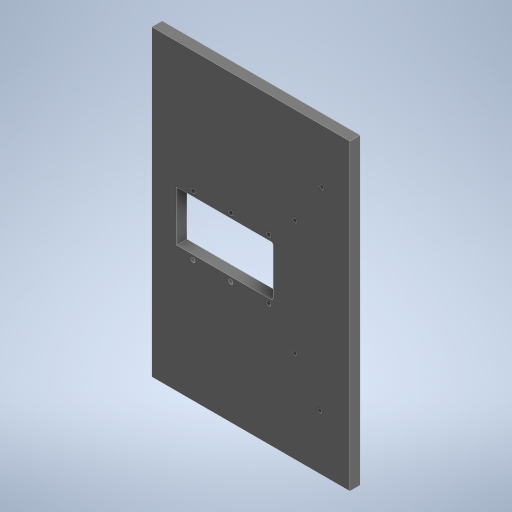
# Autodesk Inventor part: 12_CPY
Saved by Autodesk Inventor 2024.3 (Build 283343000, 343)
## iProperties
Created: 2024-09-08
Part Number: 12_CPY
Material: 아크릴, 선명
Document SubType Name: Modeling
Designer: 구지현
Mass: 132.436 g
Surface Area: 421.006 cm^2
Volume: 111.29 cm^3
Density: 1.19 g/cm^3
Appearance: 회색
Author: 구지현
Autodesk Inventor part; units mm, degrees
ref_plane "YZ Plane" through (0, 0, 0) normal (1, 0, 0) x (0, 1, 0)
ref_plane "XZ Plane" through (0, 0, 0) normal (0, 1, 0) x (-1, 0, 0)
ref_plane "XY Plane" through (0, 0, 0) normal (0, 0, 1) x (1, 0, 0)
ref_plane "작업 평면1" through (-11.501, -90.6951, 25.5) normal (0, 0, 1) x (0, 1, 0)
sketch "스케치1" plane through (-11.501, -90.6951, 25.5) normal (0, 0, 1) x (0, 1, 0)
  line L0 (-0.0049, 0) -> (27.5951, 0)
  line L1 (27.5951, 0) -> (27.5951, 6)
  line L2 (-0.0049, 6) -> (27.5951, 6)
  line L3 (-0.0049, 0) -> (-0.0049, 6)
  line L4 (127.3951, 6) -> (99.7951, 6)
  line L5 (99.7951, 6) -> (99.7951, 0)
  line L6 (127.3951, 0) -> (99.7951, 0)
  line L7 (127.3951, 6) -> (127.3951, 0)
  line L8 (99.8951, -54.101) -> (127.4951, -54.101)
  line L9 (127.4951, -54.101) -> (127.4951, -48.101)
  line L10 (99.8951, -48.101) -> (127.4951, -48.101)
  line L11 (99.8951, -54.101) -> (99.8951, -48.101)
  line L12 (27.4951, -48.101) -> (-0.1049, -48.101)
  line L13 (-0.1049, -48.101) -> (-0.1049, -54.101)
  line L14 (27.4951, -54.101) -> (-0.1049, -54.101)
  line L15 (27.4951, -48.101) -> (27.4951, -54.101)
  line L16 (-0.2463, -60.601) -> (-0.2463, -62.601)
  line L17 (-0.2463, -62.601) -> (1.1951, -62.601)
  line L18 (1.1951, -62.601) -> (1.1951, -92.601)
  line L19 (1.1951, -92.601) -> (-0.2463, -92.601)
  line L20 (-0.2463, -92.601) -> (-0.2463, -94.601)
  line L21 (-0.2463, -94.601) -> (6.0451, -94.601)
  line L22 (21.3451, -94.601) -> (6.0451, -94.601)
  line L23 (21.3451, -94.601) -> (27.6365, -94.601)
  line L24 (27.6365, -92.601) -> (27.6365, -94.601)
  line L25 (27.6365, -92.601) -> (26.1951, -92.601)
  line L26 (26.1951, -62.601) -> (26.1951, -92.601)
  line L27 (26.1951, -62.601) -> (27.6365, -62.601)
  line L28 (27.6365, -60.601) -> (27.6365, -62.601)
  line L29 (27.6365, -60.601) -> (26.6951, -60.601)
  line L30 (26.6951, -60.601) -> (26.6951, -59.101)
  line L31 (0.6951, -59.101) -> (26.6951, -59.101)
  line L32 (0.6951, -59.101) -> (0.6951, -60.601)
  line L33 (0.6951, -60.601) -> (-0.2463, -60.601)
  line L34 (35.6951, -14.501) -> (35.6951, -37.501)
  line L35 (35.6951, -14.501) -> (30.6951, -14.501)
  line L36 (30.6951, -14.501) -> (30.6951, -11.001)
  line L37 (28.6951, -11.001) -> (30.6951, -11.001)
  line L38 (28.6951, -11.001) -> (28.6951, -13.501)
  line L39 (28.6951, -13.501) -> (-1.3049, -13.501)
  line L40 (-1.3049, -13.501) -> (-1.3049, -11.001)
  line L41 (-1.3049, -11.001) -> (-3.3049, -11.001)
  line L42 (-3.3049, -11.001) -> (-3.3049, -16.751)
  line L43 (-5.8049, -16.751) -> (-3.3049, -16.751)
  spline S0 degree 3 poles (-5.8049, -16.751) (-6.0293, -16.751) (-6.2964, -16.7855) (-6.6655, -16.908) (-6.8416, -16.9972) (-7.0685, -17.1834) (-7.1685, -17.3017) (-7.2736, -17.5152) (-7.3049, -17.6421) (-7.3049, -17.751) knots 0 0 0 0 0.358 0.358 0.620378 0.620378 0.826274 0.826274 1 1 1 1
  line L44 (-7.3049, -34.251) -> (-7.3049, -17.751)
  spline S1 degree 3 poles (-7.3049, -34.251) (-7.3049, -34.3599) (-7.2736, -34.4868) (-7.1685, -34.7003) (-7.0685, -34.8186) (-6.8416, -35.0048) (-6.6655, -35.094) (-6.2964, -35.2165) (-6.0293, -35.251) (-5.8049, -35.251) knots 0 0 0 0 0.173726 0.173726 0.379622 0.379622 0.642 0.642 1 1 1 1
  line L45 (-5.8049, -35.251) -> (-3.3049, -35.251)
  line L46 (-3.3049, -35.251) -> (-3.3049, -41.001)
  line L47 (-1.3049, -41.001) -> (-3.3049, -41.001)
  line L48 (-1.3049, -41.001) -> (-1.3049, -38.501)
  line L49 (28.6951, -38.501) -> (-1.3049, -38.501)
  line L50 (28.6951, -38.501) -> (28.6951, -41.001)
  line L51 (28.6951, -41.001) -> (30.6951, -41.001)
  line L52 (30.6951, -41.001) -> (30.6951, -37.501)
  line L53 (35.6951, -37.501) -> (30.6951, -37.501)
  line L54 (135.6951, -14.501) -> (135.6951, -37.501)
  line L55 (135.6951, -14.501) -> (130.6951, -14.501)
  line L56 (130.6951, -14.501) -> (130.6951, -11.001)
  line L57 (128.6951, -11.001) -> (130.6951, -11.001)
  line L58 (128.6951, -11.001) -> (128.6951, -13.501)
  line L59 (128.6951, -13.501) -> (98.6951, -13.501)
  line L60 (98.6951, -13.501) -> (98.6951, -11.001)
  line L61 (98.6951, -11.001) -> (96.6951, -11.001)
  line L62 (96.6951, -11.001) -> (96.6951, -16.751)
  line L63 (94.1951, -16.751) -> (96.6951, -16.751)
  spline S2 degree 3 poles (94.1951, -16.751) (93.9707, -16.751) (93.7036, -16.7855) (93.3345, -16.908) (93.1584, -16.9972) (92.9315, -17.1834) (92.8315, -17.3017) (92.7264, -17.5152) (92.6951, -17.6421) (92.6951, -17.751) knots 0 0 0 0 0.358 0.358 0.620378 0.620378 0.826274 0.826274 1 1 1 1
  line L64 (92.6951, -34.251) -> (92.6951, -17.751)
  spline S3 degree 3 poles (92.6951, -34.251) (92.6951, -34.3599) (92.7264, -34.4868) (92.8315, -34.7003) (92.9315, -34.8186) (93.1584, -35.0048) (93.3345, -35.094) (93.7036, -35.2165) (93.9707, -35.251) (94.1951, -35.251) knots 0 0 0 0 0.173726 0.173726 0.379622 0.379622 0.642 0.642 1 1 1 1
  line L65 (94.1951, -35.251) -> (96.6951, -35.251)
  line L66 (96.6951, -35.251) -> (96.6951, -41.001)
  line L67 (98.6951, -41.001) -> (96.6951, -41.001)
  line L68 (98.6951, -41.001) -> (98.6951, -38.501)
  line L69 (128.6951, -38.501) -> (98.6951, -38.501)
  line L70 (128.6951, -38.501) -> (128.6951, -41.001)
  line L71 (128.6951, -41.001) -> (130.6951, -41.001)
  line L72 (130.6951, -41.001) -> (130.6951, -37.501)
  line L73 (135.6951, -37.501) -> (130.6951, -37.501)
  line L74 (99.7537, -60.601) -> (99.7537, -62.601)
  line L75 (99.7537, -62.601) -> (101.1951, -62.601)
  line L76 (101.1951, -62.601) -> (101.1951, -92.601)
  line L77 (101.1951, -92.601) -> (99.7537, -92.601)
  line L78 (99.7537, -92.601) -> (99.7537, -94.601)
  line L79 (99.7537, -94.601) -> (106.0451, -94.601)
  line L80 (121.3451, -94.601) -> (106.0451, -94.601)
  line L81 (121.3451, -94.601) -> (127.6365, -94.601)
  line L82 (127.6365, -92.601) -> (127.6365, -94.601)
  line L83 (127.6365, -92.601) -> (126.1951, -92.601)
  line L84 (126.1951, -62.601) -> (126.1951, -92.601)
  line L85 (126.1951, -62.601) -> (127.6365, -62.601)
  line L86 (127.6365, -60.601) -> (127.6365, -62.601)
  line L87 (127.6365, -60.601) -> (126.6951, -60.601)
  line L88 (126.6951, -60.601) -> (126.6951, -59.101)
  line L89 (100.6951, -59.101) -> (126.6951, -59.101)
  line L90 (100.6951, -59.101) -> (100.6951, -60.601)
  line L91 (100.6951, -60.601) -> (99.7537, -60.601)
  line L92 (21.3451, 6) -> (21.3451, 12)
  line L93 (1.1951, -62.601) -> (1.1951, 11.399)
  line L94 (-24.3049, -26.001) -> (-24.3049, -76.001)
  line L95 (-24.3049, -76.001) -> (-18.3049, -76.001)
  line L96 (-18.3049, -26.001) -> (-18.3049, -76.001)
  line L97 (-24.3049, -26.001) -> (-18.3049, -26.001)
  line L98 (145.6951, -26.001) -> (145.6951, -76.001)
  line L99 (145.6951, -76.001) -> (151.6951, -76.001)
  line L100 (151.6951, -26.001) -> (151.6951, -76.001)
  line L101 (145.6951, -26.001) -> (151.6951, -26.001)
  line L102 (-24.3049, -52.5323) -> (151.6951, -52.5323)
  line L103 (1.1951, 11.399) -> (-33.5056, 11.399)
  line L104 (1.1951, -62.601) -> (-24.3049, -62.601)
  line L105 (-24.3049, -62.601) -> (151.6951, -62.601)
  line L106 (151.6951, -62.601) -> (151.6951, 11.399)
  line L107 (151.6951, 11.399) -> (-24.3049, 11.399)
  line L108 (-24.3049, 11.399) -> (-24.3049, -62.601)
  circle A0 centre (-0.0049, 0) radius 1
  circle A1 centre (-0.0049, 6) radius 1
  circle A2 centre (27.5951, 6) radius 1
  circle A3 centre (27.5951, 0) radius 1
  circle A4 centre (99.7951, 0) radius 1
  circle A5 centre (99.7951, 6) radius 1
  circle A6 centre (127.3951, 6) radius 1
  circle A7 centre (127.3951, 0) radius 1
  circle A8 centre (99.8951, -54.101) radius 1
  circle A9 centre (99.8951, -48.101) radius 1
  circle A10 centre (127.4951, -48.101) radius 1
  circle A11 centre (127.6365, -54.101) radius 1
  circle A12 centre (27.4951, -54.101) radius 1
  circle A13 centre (27.5951, -48.101) radius 1
  circle A14 centre (-0.1049, -48.101) radius 1
  circle A15 centre (-0.1049, -54.101) radius 1
  point P0 (90.6951, -11.501)
  point P1 (99.8951, -49.101)
  point P2 (100.8951, -48.101)
  point P3 (126.4951, -48.101)
  point P4 (127.4951, -49.101)
  point P5 (127.4951, -53.1111)
  point P6 (126.6365, -54.101)
  point P7 (100.8951, -54.101)
  point P8 (99.8951, -53.101)
  point P9 (126.3951, 0)
  point P10 (100.7951, 0)
  point P11 (99.7951, 1)
  point P12 (99.7951, 5)
  point P13 (100.7951, 6)
  point P14 (126.3951, 6)
  point P15 (127.3951, 5)
  point P16 (127.3951, 1)
  point P17 (26.5951, 6)
  point P18 (27.5951, 5)
  point P19 (27.5951, 1)
  point P20 (26.5951, 0)
  point P21 (0.9951, 0)
  point P22 (-0.0049, 1)
  point P23 (-0.0049, 5)
  point P24 (0.9951, 6)
  point P25 (26.5951, -48.101)
  point P26 (27.4951, -49.096)
  point P27 (27.4951, -53.101)
  point P28 (26.4951, -54.101)
  point P29 (0.8951, -54.101)
  point P30 (-0.1049, -53.101)
  point P31 (-0.1049, -49.101)
  point P32 (0.8951, -48.101)
  point P33 (-0.2463, -62.601)
  point P34 (1.1951, -62.601)
  point P35 (99.7537, -62.601)
  point P36 (101.1951, -62.601)
  point P37 (126.1951, -62.601)
  point P38 (127.6365, -62.601)
  point P39 (151.6951, -62.601)
  point P40 (1.1951, 11.399)
  point P41 (-24.3049, 11.399)
  dimension "d0" = 6
  dimension "d1" = 74
  dimension "d2" = 2
  dimension "d3" = 2
  dimension "d4" = 2
  dimension "d5" = 2
  dimension "d6" = 2
  dimension "d7" = 2
  dimension "d8" = 2
  dimension "d9" = 2
  dimension "d10" = 2
  dimension "d11" = 2
  dimension "d12" = 2
  dimension "d13" = 2
  dimension "d14" = 2
  dimension "d15" = 2
  dimension "d16" = 2
  dimension "d17" = 2
  constraints: 18 end point, 16 centre point, 14 coincident, 4 point on line, 3 perpendicular, 2 horizontal, 2 parallel, 2 vertical
  measures "d0" distance of L92.start L92.end
  measures "d1" distance of L17.end L93.end
  measures "d2" diameter of A0
  measures "d3" diameter of A1
  measures "d4" diameter of A2
  measures "d5" diameter of A3
  measures "d6" diameter of A4
  measures "d7" diameter of A5
  measures "d8" diameter of A6
  measures "d9" diameter of A7
  measures "d10" diameter of A8
  measures "d11" diameter of A9
  measures "d12" diameter of A10
  measures "d13" diameter of A11
  measures "d14" diameter of A12
  measures "d15" diameter of A13
  measures "d16" diameter of A14
  measures "d17" diameter of A15
extrude "돌출1" add sketch "스케치1" along normal blind 6 contours L0 L93 L39 L40 L41 L42 L43 S0 L44 S1 L45 L46 L47 L48 L49 L12 A14 L13 L102 L96 L97 L108 L103 L2 A1 L3 A0 | L0 A3 L1 A2 L2 L92 L107 L106 L101 L98 L102 L9 A10 L10 A9 L11 L15 A13 L12 L93 L49 L50 L51 L52 L53 L34 L35 L36 L37 L38 L39 | L93 L49 L48 L47 L46 L45 S1 L44 S0 L43 L42 L41 L40 L39 | L39 L38 L37 L36 L35 L34 L53 L52 L51 L50 L49 L93 | L93 L107 L92 L2 | L97 L96 L102 L94 | L93 L31 L32 L33 L16 L104 L96 L102 L13 A15 L14 | L14 A12 L15 L102 L11 A8 L8 A11 L9 L98 L105 L86 L87 L88 L89 L90 L91 L74 L28 L29 L30 L31 L93 | L100 L102 L98 L101 | L102 L96 L104 L94 | L93 L17 L16 L33 L32 L31 | L31 L30 L29 L28 L27 L105 L93 | L100 L105 L98 L102 | L85 L105 L75 L74 L91 L90 L89 L88 L87 L86 | L54 L73 L72 L71 L70 L69 L68 L67 L66 L65 S3 L64 S2 L63 L62 L61 L60 L59 L58 L57 L56 L55
sketch "스케치3" plane through (-11.501, -90.6951, 31.5) normal (0, 0, 1) x (1, 0, 0)
  line L0 (-11.399, 151.6951) -> (-11.399, -24.3049) projected
  line L1 (-11.399, 151.6951) -> (-11.399, 63.6951)
  line L2 (62.601, -24.3049) -> (62.601, 151.6951) projected
  line L3 (62.601, 151.6951) -> (-11.399, 151.6951) projected
  line L4 (-11.399, 151.6951) -> (-11.399, -24.3049) projected
  line L5 (-11.399, -24.3049) -> (62.601, -24.3049) projected
  line L6 (53.101, 99.8951) -> (49.101, 99.8951) projected
  arc A0 (48.101, 100.8951) -> (49.101, 99.8951) centre (48.101, 99.8951) ccw projected
  line L7 (48.101, 100.8951) -> (48.101, 126.4951) projected
  arc A1 (49.101, 127.4951) -> (48.101, 126.4951) centre (48.101, 127.4951) ccw projected
  line L8 (49.101, 127.4951) -> (53.1111, 127.4951) projected
  arc A2 (54.101, 126.6365) -> (53.1111, 127.4951) centre (54.101, 127.6365) ccw projected
  line L9 (54.101, 126.6365) -> (54.101, 100.8951) projected
  arc A3 (53.101, 99.8951) -> (54.101, 100.8951) centre (54.101, 99.8951) ccw projected
  arc A4 (0, 126.3951) -> (-1, 127.3951) centre (0, 127.3951) ccw projected
  line L10 (0, 126.3951) -> (0, 100.7951) projected
  arc A5 (-1, 99.7951) -> (0, 100.7951) centre (0, 99.7951) ccw projected
  line L11 (-1, 99.7951) -> (-5, 99.7951) projected
  arc A6 (-6, 100.7951) -> (-5, 99.7951) centre (-6, 99.7951) ccw projected
  line L12 (-6, 100.7951) -> (-6, 126.3951) projected
  arc A7 (-5, 127.3951) -> (-6, 126.3951) centre (-6, 127.3951) ccw projected
  line L13 (-5, 127.3951) -> (-1, 127.3951) projected
  line L14 (-6, 0.9951) -> (-6, 26.5951) projected
  arc A8 (-5, 27.5951) -> (-6, 26.5951) centre (-6, 27.5951) ccw projected
  line L15 (-5, 27.5951) -> (-1, 27.5951) projected
  arc A9 (0, 26.5951) -> (-1, 27.5951) centre (0, 27.5951) ccw projected
  line L16 (0, 26.5951) -> (0, 0.9951) projected
  arc A10 (-1, -0.0049) -> (0, 0.9951) centre (0, -0.0049) ccw projected
  line L17 (-1, -0.0049) -> (-5, -0.0049) projected
  arc A11 (-6, 0.9951) -> (-5, -0.0049) centre (-6, -0.0049) ccw projected
  line L18 (48.101, 0.8951) -> (48.101, 26.5951) projected
  arc A12 (49.096, 27.4951) -> (48.101, 26.5951) centre (48.101, 27.5951) ccw projected
  line L19 (49.096, 27.4951) -> (53.101, 27.4951) projected
  arc A13 (54.101, 26.4951) -> (53.101, 27.4951) centre (54.101, 27.4951) ccw projected
  line L20 (54.101, 26.4951) -> (54.101, 0.8951) projected
  arc A14 (53.101, -0.1049) -> (54.101, 0.8951) centre (54.101, -0.1049) ccw projected
  line L21 (53.101, -0.1049) -> (49.101, -0.1049) projected
  arc A15 (48.101, 0.8951) -> (49.101, -0.1049) centre (48.101, -0.1049) ccw projected
  line L22 (-11.399, 63.6951) -> (62.601, 63.6951)
  circle A16 centre (-0.5531, 64.2887) radius 1.55 projected
  circle A17 centre (11.0245, 74.6791) radius 1.55 projected
  circle A18 centre (21.4149, 63.1016) radius 1.55 projected
  circle A19 centre (9.8373, 52.7111) radius 1.55 projected
  circle A20 centre (10.4309, 63.6951) radius 5 projected
  circle A21 centre (10.4309, 63.6951) radius 13.9 projected
  circle A22 centre (17.778, 55.5086) radius 1.55 projected
  circle A23 centre (18.6175, 71.0422) radius 1.55 projected
  circle A24 centre (3.0838, 71.8817) radius 1.55 projected
  circle A25 centre (2.2443, 56.348) radius 1.55 projected
  circle A26 centre (3.0838, 71.8817) radius 1.65
  circle A27 centre (-0.5531, 64.2887) radius 1.65
  circle A28 centre (2.2443, 56.348) radius 1.65
  circle A29 centre (9.8373, 52.7111) radius 1.65
  circle A30 centre (17.778, 55.5086) radius 1.65
  circle A31 centre (21.4149, 63.1016) radius 1.65
  circle A32 centre (18.6175, 71.0422) radius 1.65
  circle A33 centre (11.0245, 74.6791) radius 1.65
  circle A34 centre (10.4309, 63.6951) radius 5.1
  point P0 (11.501, 90.6951)
  dimension "d32" = 88
  dimension "d33" = 0.1
  dimension "d34" = 0.1
  dimension "d35" = 0.1
  dimension "d36" = 0.1
  dimension "d37" = 0.1
  dimension "d38" = 0.1
  dimension "d39" = 0.1
  dimension "d40" = 0.1
  dimension "d41" = 0.1
  constraints: 9 centre point, 4 end point, 2 midpoint
  measures "d32" distance of L0.start L1.end
  measures "d33" radial gap between concentric circles of A24 A26
  measures "d34" radial gap between concentric circles of A16 A27
  measures "d35" radial gap between concentric circles of A25 A28
  measures "d36" radial gap between concentric circles of A19 A29
  measures "d37" radial gap between concentric circles of A22 A30
  measures "d38" radial gap between concentric circles of A18 A31
  measures "d39" radial gap between concentric circles of A23 A32
  measures "d40" radial gap between concentric circles of A17 A33
  measures "d41" radial gap between concentric circles of A20 A34
extrude "돌출3" cut sketch "스케치3" against normal blind 10 contours A16 L22 | L22 A16 | A31 L22 A18 | L22 A18 A31 | A34 L22 A20 | L22 A20 A34 | A18 L22 | L22 A18 | A20 L22 | L22 A20 | A17 | A19 | A22 | A23 | A24 | A25 | A26 | A28 | A29 | A30 | A32 | A33
sketch "스케치4" plane through (-22.9, -115, 25.5) normal (-1, 0, 0) x (0, 0, 1)
  line L0 (0, 176) -> (0, 0) projected
  line L1 (0, 0) -> (6, 0) projected
  line L2 (6, 176) -> (6, 0) projected
  line L3 (0, 176) -> (6, 176) projected
  line L4 (74, 151) -> (80, 151) projected
  line L5 (80, 151) -> (80, 176) projected
  line L6 (80, 176) -> (0, 176) projected
  line L7 (0, 176) -> (0, 151) projected
  line L8 (0, 151) -> (6, 151) projected
  line L9 (6, 151) -> (6, 109) projected
  line L10 (6, 109) -> (0, 109) projected
  line L11 (0, 109) -> (0, 67) projected
  line L12 (0, 67) -> (6, 67) projected
  line L13 (6, 67) -> (6, 25) projected
  line L14 (6, 25) -> (0, 25) projected
  line L15 (0, 25) -> (0, 0) projected
  line L16 (0, 0) -> (80, 0) projected
  line L17 (80, 0) -> (80, 25) projected
  line L18 (80, 25) -> (74, 25) projected
  line L19 (74, 25) -> (74, 67) projected
  line L20 (74, 67) -> (80, 67) projected
  line L21 (80, 67) -> (80, 109) projected
  line L22 (80, 109) -> (74, 109) projected
  line L23 (74, 109) -> (74, 151) projected
  line L24 (60, 156) -> (60, 25) projected
  line L25 (60, 25) -> (20, 25) projected
  line L26 (20, 25) -> (20, 156) projected
  line L27 (20, 156) -> (60, 156) projected
  point P0 (-25.5, 115)
extrude "돌출4" add sketch "스케치4" along normal blind 6 contours L8 L2 L10 L0 | L12 L2 L14 L0
sketch "스케치5" plane through (51.1, -115, 25.5) normal (1, 0, 0) x (0, 0, -1)
  line L0 (0, 0) -> (0, 176) projected
  line L1 (0, 176) -> (-6, 176) projected
  line L2 (-6, 0) -> (-6, 176) projected
  line L3 (0, 0) -> (-6, 0) projected
  line L4 (-74, 151) -> (-80, 151) projected
  line L5 (-74, 109) -> (-74, 151) projected
  line L6 (-80, 109) -> (-74, 109) projected
  line L7 (-80, 67) -> (-80, 109) projected
  line L8 (-74, 67) -> (-80, 67) projected
  line L9 (-74, 25) -> (-74, 67) projected
  line L10 (-80, 25) -> (-74, 25) projected
  line L11 (-80, 0) -> (-80, 25) projected
  line L12 (0, 0) -> (-80, 0) projected
  line L13 (0, 25) -> (0, 0) projected
  line L14 (-6, 25) -> (0, 25) projected
  line L15 (-6, 67) -> (-6, 25) projected
  line L16 (0, 67) -> (-6, 67) projected
  line L17 (0, 109) -> (0, 67) projected
  line L18 (-6, 109) -> (0, 109) projected
  line L19 (-6, 151) -> (-6, 109) projected
  line L20 (0, 151) -> (-6, 151) projected
  line L21 (0, 176) -> (0, 151) projected
  line L22 (-80, 176) -> (0, 176) projected
  line L23 (-80, 151) -> (-80, 176) projected
  line L24 (-60, 156) -> (-60, 25) projected
  line L25 (-20, 156) -> (-60, 156) projected
  line L26 (-20, 25) -> (-20, 156) projected
  line L27 (-60, 25) -> (-20, 25) projected
  point P0 (25.5, 115)
extrude "돌출5" cut sketch "스케치5" against normal blind 6 contours L3 L2 L14 L0 | L16 L2 L18 L0 | L20 L2 L1 L0
move faces "이동1" translate (5, 0, 0) faces at (45.1, -20, 29.5) (45.1, -106.6667, 27.5) (51.1, -58.0391, 27.5) (51.1, -72.0391, 27.5) (51.1, 27.0195, 29.5) (51.1, -0.9805, 27.5) (47.1, -6, 27.5) (49.1, -48, 29.5) (47.1, -90, 27.5) (45.1, 44.3333, 27.5)
sketch "스케치6" plane through (-22.9, -115, 25.5) normal (0, -1, 0) x (1, 0, 0)
  line L0 (0, 20) -> (0, 6) projected
  line L1 (0, 6) -> (9, 6) projected
  line L2 (9, 6) -> (9, 0) projected
  line L3 (9, 0) -> (29, 0) projected
  line L4 (29, 0) -> (29, 6) projected
  line L5 (29, 6) -> (44, 6) projected
  line L6 (44, 6) -> (44, 0) projected
  line L7 (44, 0) -> (64, 0) projected
  line L8 (64, 0) -> (64, 6) projected
  line L9 (64, 6) -> (73, 6) projected
  line L10 (73, 6) -> (73, 20) projected
  line L11 (73, 20) -> (79, 20) projected
  line L12 (79, 20) -> (79, 60) projected
  line L13 (79, 60) -> (73, 60) projected
  line L14 (73, 60) -> (73, 80) projected
  line L15 (73, 80) -> (64, 80) projected
  line L16 (64, 80) -> (64, 74) projected
  line L17 (64, 74) -> (44, 74) projected
  line L18 (44, 74) -> (44, 80) projected
  line L19 (44, 80) -> (29, 80) projected
  line L20 (29, 80) -> (29, 74) projected
  line L21 (29, 74) -> (9, 74) projected
  line L22 (9, 74) -> (9, 80) projected
  line L23 (9, 80) -> (0, 80) projected
  line L24 (0, 80) -> (0, 60) projected
  line L25 (0, 60) -> (-6, 60) projected
  line L26 (-6, 60) -> (-6, 20) projected
  line L27 (-6, 20) -> (0, 20) projected
  line L28 (0, 0) -> (0, 80) projected
  line L29 (0, 80) -> (-6, 80) projected
  line L30 (-6, 0) -> (-6, 80) projected
  line L31 (0, 0) -> (-6, 0) projected
  line L32 (79, 0) -> (79, 80) projected
  line L33 (79, 80) -> (73, 80) projected
  line L34 (73, 0) -> (73, 80) projected
  line L35 (79, 0) -> (73, 0) projected
  line L36 (73, 0) -> (73, 6) projected
  line L37 (0, 6) -> (73, 6) projected
  line L38 (0, 0) -> (0, 6) projected
  line L39 (0, 0) -> (73, 0) projected
  point P0 (22.9, -25.5)
  point P1 (64, 6)
  point P2 (44, 6)
  point P3 (29, 6)
  point P4 (9, 6)
extrude "돌출6" cut sketch "스케치6" against normal blind 6 contours L37 L4 L3 L2 | L37 L8 L7 L6
sketch "스케치7" plane through (-11.501, -90.6951, 31.5) normal (0, 0, 1) x (1, 0, 0)
  line L0 (-2.399, 151.6951) -> (-2.399, 145.6951) projected
  line L1 (-2.399, 145.6951) -> (-11.399, 145.6951) projected
  line L2 (-11.399, 145.6951) -> (-11.399, 126.6951) projected
  line L3 (-11.399, 126.6951) -> (-17.399, 126.6951) projected
  line L4 (-17.399, 84.6951) -> (-17.399, 126.6951) projected
  line L5 (-11.399, 84.6951) -> (-17.399, 84.6951) projected
  line L6 (-11.399, 84.6951) -> (-11.399, 42.6951) projected
  line L7 (-11.399, 42.6951) -> (-17.399, 42.6951) projected
  line L8 (-17.399, 0.6951) -> (-17.399, 42.6951) projected
  line L9 (-11.399, 0.6951) -> (-17.399, 0.6951) projected
  line L10 (-11.399, 0.6951) -> (-11.399, -18.3049) projected
  line L11 (-11.399, -18.3049) -> (-2.399, -18.3049) projected
  line L12 (-2.399, -18.3049) -> (-2.399, -24.3049) projected
  line L13 (-2.399, -24.3049) -> (17.601, -24.3049) projected
  line L14 (17.601, -24.3049) -> (17.601, -18.3049) projected
  line L15 (17.601, -18.3049) -> (32.601, -18.3049) projected
  line L16 (32.601, -18.3049) -> (32.601, -24.3049) projected
  line L17 (32.601, -24.3049) -> (52.601, -24.3049) projected
  line L18 (52.601, -24.3049) -> (52.601, -18.3049) projected
  line L19 (52.601, -18.3049) -> (61.601, -18.3049) projected
  line L20 (61.601, -18.3049) -> (61.601, 0.6951) projected
  line L21 (61.601, 0.6951) -> (67.601, 0.6951) projected
  line L22 (67.601, 0.6951) -> (67.601, 42.6951) projected
  line L23 (67.601, 42.6951) -> (61.601, 42.6951) projected
  line L24 (61.601, 42.6951) -> (61.601, 84.6951) projected
  line L25 (61.601, 84.6951) -> (67.601, 84.6951) projected
  line L26 (67.601, 84.6951) -> (67.601, 126.6951) projected
  line L27 (67.601, 126.6951) -> (61.601, 126.6951) projected
  line L28 (61.601, 126.6951) -> (61.601, 145.6951) projected
  line L29 (61.601, 145.6951) -> (52.601, 145.6951) projected
  line L30 (52.601, 145.6951) -> (52.601, 151.6951) projected
  line L31 (52.601, 151.6951) -> (32.601, 151.6951) projected
  line L32 (32.601, 151.6951) -> (32.601, 145.6951) projected
  line L33 (32.601, 145.6951) -> (17.601, 145.6951) projected
  line L34 (17.601, 145.6951) -> (17.601, 151.6951) projected
  line L35 (17.601, 151.6951) -> (-2.399, 151.6951) projected
  line L36 (52.601, -18.3049) -> (52.601, -24.3049) projected
  line L37 (52.601, -24.3049) -> (61.601, -24.3049) projected
  line L38 (61.601, -24.3049) -> (61.601, 0.6951) projected
  line L39 (61.601, 0.6951) -> (67.601, 0.6951) projected
  line L40 (67.601, 0.6951) -> (67.601, 42.6951) projected
  line L41 (67.601, 42.6951) -> (61.601, 42.6951) projected
  line L42 (61.601, 42.6951) -> (61.601, 84.6951) projected
  line L43 (61.601, 84.6951) -> (67.601, 84.6951) projected
  line L44 (67.601, 84.6951) -> (67.601, 126.6951) projected
  line L45 (67.601, 126.6951) -> (61.601, 126.6951) projected
  line L46 (61.601, 126.6951) -> (61.601, 151.6951) projected
  line L47 (61.601, 151.6951) -> (-11.399, 151.6951) projected
  line L48 (-11.399, 151.6951) -> (-11.399, 126.6951) projected
  line L49 (-11.399, 126.6951) -> (-17.399, 126.6951) projected
  line L50 (-17.399, 84.6951) -> (-17.399, 126.6951) projected
  line L51 (-11.399, 84.6951) -> (-17.399, 84.6951) projected
  line L52 (-11.399, 84.6951) -> (-11.399, 42.6951) projected
  line L53 (-11.399, 42.6951) -> (-17.399, 42.6951) projected
  line L54 (-17.399, 0.6951) -> (-17.399, 42.6951) projected
  line L55 (-11.399, 0.6951) -> (-17.399, 0.6951) projected
  line L56 (-11.399, 0.6951) -> (-11.399, -24.3049) projected
  line L57 (-11.399, -24.3049) -> (-2.399, -24.3049) projected
  line L58 (-2.399, -24.3049) -> (-2.399, -18.3049) projected
  line L59 (-2.399, -18.3049) -> (17.601, -18.3049) projected
  line L60 (17.601, -18.3049) -> (17.601, -24.3049) projected
  line L61 (17.601, -24.3049) -> (32.601, -24.3049) projected
  line L62 (32.601, -24.3049) -> (32.601, -18.3049) projected
  line L63 (32.601, -18.3049) -> (52.601, -18.3049) projected
  circle A0 centre (-0.5531, 64.2887) radius 1.55 projected
  circle A1 centre (17.778, 55.5086) radius 1.65 projected
  circle A2 centre (21.4149, 63.1016) radius 1.65 projected
  circle A3 centre (10.4309, 63.6951) radius 5.1 projected
  circle A4 centre (3.0838, 71.8817) radius 1.65 projected
  circle A5 centre (9.8373, 52.7111) radius 1.65 projected
  circle A6 centre (18.6175, 71.0422) radius 1.65 projected
  circle A7 centre (2.2443, 56.348) radius 1.65 projected
  circle A8 centre (11.0245, 74.6791) radius 1.65 projected
  line L64 (53.101, 99.8951) -> (49.101, 99.8951) projected
  arc A9 (48.101, 100.8951) -> (49.101, 99.8951) centre (48.101, 99.8951) ccw projected
  line L65 (48.101, 100.8951) -> (48.101, 126.4951) projected
  arc A10 (49.101, 127.4951) -> (48.101, 126.4951) centre (48.101, 127.4951) ccw projected
  line L66 (49.101, 127.4951) -> (53.1111, 127.4951) projected
  arc A11 (54.101, 126.6365) -> (53.1111, 127.4951) centre (54.101, 127.6365) ccw projected
  line L67 (54.101, 126.6365) -> (54.101, 100.8951) projected
  arc A12 (53.101, 99.8951) -> (54.101, 100.8951) centre (54.101, 99.8951) ccw projected
  arc A13 (0, 126.3951) -> (-1, 127.3951) centre (0, 127.3951) ccw projected
  line L68 (0, 126.3951) -> (0, 100.7951) projected
  arc A14 (-1, 99.7951) -> (0, 100.7951) centre (0, 99.7951) ccw projected
  line L69 (-1, 99.7951) -> (-5, 99.7951) projected
  arc A15 (-6, 100.7951) -> (-5, 99.7951) centre (-6, 99.7951) ccw projected
  line L70 (-6, 100.7951) -> (-6, 126.3951) projected
  arc A16 (-5, 127.3951) -> (-6, 126.3951) centre (-6, 127.3951) ccw projected
  line L71 (-5, 127.3951) -> (-1, 127.3951) projected
  line L72 (-6, 0.9951) -> (-6, 26.5951) projected
  arc A17 (-5, 27.5951) -> (-6, 26.5951) centre (-6, 27.5951) ccw projected
  line L73 (-5, 27.5951) -> (-1, 27.5951) projected
  arc A18 (0, 26.5951) -> (-1, 27.5951) centre (0, 27.5951) ccw projected
  line L74 (0, 26.5951) -> (0, 0.9951) projected
  arc A19 (-1, -0.0049) -> (0, 0.9951) centre (0, -0.0049) ccw projected
  line L75 (-1, -0.0049) -> (-5, -0.0049) projected
  arc A20 (-6, 0.9951) -> (-5, -0.0049) centre (-6, -0.0049) ccw projected
  line L76 (48.101, 0.8951) -> (48.101, 26.5951) projected
  arc A21 (49.096, 27.4951) -> (48.101, 26.5951) centre (48.101, 27.5951) ccw projected
  line L77 (49.096, 27.4951) -> (53.101, 27.4951) projected
  arc A22 (54.101, 26.4951) -> (53.101, 27.4951) centre (54.101, 27.4951) ccw projected
  line L78 (54.101, 26.4951) -> (54.101, 0.8951) projected
  arc A23 (53.101, -0.1049) -> (54.101, 0.8951) centre (54.101, -0.1049) ccw projected
  line L79 (53.101, -0.1049) -> (49.101, -0.1049) projected
  arc A24 (48.101, 0.8951) -> (49.101, -0.1049) centre (48.101, -0.1049) ccw projected
  line L80 (-2.399, 151.6951) -> (-2.399, 145.6951) projected
  line L81 (-2.399, 145.6951) -> (-11.399, 145.6951) projected
  line L82 (-11.399, 145.6951) -> (-11.399, 126.6951) projected
  line L83 (-11.399, 126.6951) -> (-17.399, 126.6951) projected
  line L84 (-17.399, 84.6951) -> (-17.399, 126.6951) projected
  line L85 (-11.399, 84.6951) -> (-17.399, 84.6951) projected
  line L86 (-11.399, 84.6951) -> (-11.399, 42.6951) projected
  line L87 (-11.399, 42.6951) -> (-17.399, 42.6951) projected
  line L88 (-17.399, 0.6951) -> (-17.399, 42.6951) projected
  line L89 (-11.399, 0.6951) -> (-17.399, 0.6951) projected
  line L90 (-11.399, 0.6951) -> (-11.399, -18.3049) projected
  line L91 (-11.399, -18.3049) -> (-2.399, -18.3049) projected
  line L92 (-2.399, -18.3049) -> (-2.399, -24.3049) projected
  line L93 (-2.399, -24.3049) -> (17.601, -24.3049) projected
  line L94 (17.601, -24.3049) -> (17.601, -18.3049) projected
  line L95 (17.601, -18.3049) -> (32.601, -18.3049) projected
  line L96 (32.601, -18.3049) -> (32.601, -24.3049) projected
  line L97 (32.601, -24.3049) -> (52.601, -24.3049) projected
  line L98 (52.601, -24.3049) -> (52.601, -18.3049) projected
  line L99 (52.601, -18.3049) -> (61.601, -18.3049) projected
  line L100 (61.601, -18.3049) -> (61.601, 0.6951) projected
  line L101 (61.601, 0.6951) -> (67.601, 0.6951) projected
  line L102 (67.601, 0.6951) -> (67.601, 42.6951) projected
  line L103 (67.601, 42.6951) -> (61.601, 42.6951) projected
  line L104 (61.601, 42.6951) -> (61.601, 84.6951) projected
  line L105 (61.601, 84.6951) -> (67.601, 84.6951) projected
  line L106 (67.601, 84.6951) -> (67.601, 126.6951) projected
  line L107 (67.601, 126.6951) -> (61.601, 126.6951) projected
  line L108 (61.601, 126.6951) -> (61.601, 145.6951) projected
  line L109 (61.601, 145.6951) -> (52.601, 145.6951) projected
  line L110 (52.601, 145.6951) -> (52.601, 151.6951) projected
  line L111 (52.601, 151.6951) -> (32.601, 151.6951) projected
  line L112 (32.601, 151.6951) -> (32.601, 145.6951) projected
  line L113 (32.601, 145.6951) -> (17.601, 145.6951) projected
  line L114 (17.601, 145.6951) -> (17.601, 151.6951) projected
  line L115 (17.601, 151.6951) -> (-2.399, 151.6951) projected
  line L116 (61.601, 145.6951) -> (-11.399, 145.6951)
  line L117 (-11.399, 145.6951) -> (-11.399, 151.6951)
  line L118 (-11.399, 151.6951) -> (61.601, 151.6951)
  line L119 (61.601, 151.6951) -> (61.601, 145.6951)
  point P0 (11.501, 90.6951)
  point P1 (-11.399, 145.6951)
  point P2 (-2.399, 151.6951)
  point P3 (52.601, 151.6951)
  point P4 (61.601, 145.6951)
  point P5 (-2.399, 145.6951)
  point P6 (32.601, 145.6951)
  constraints: 8 end point, 2 parallel, 1 horizontal, 1 perpendicular
extrude "돌출7" cut sketch "스케치7" against normal blind 6 contours L35 L34 L116 L0 | L31 L30 L116 L32
sketch "스케치8" plane through (-11.501, -90.6951, 31.5) normal (0, 0, 1) x (1, 0, 0)
  arc A0 (4.1673, 44.1143) -> (5.8543, 43.5951) centre (5.8543, 46.5951) ccw projected
  line L0 (4.1673, 44.1143) -> (-1.6937, 48.0999) projected
  arc A1 (-2.5691, 49.7537) -> (-1.6937, 48.0999) centre (-0.5691, 49.7537) ccw projected
  line L1 (-2.5691, 50.6951) -> (-2.5691, 49.7537) projected
  arc A2 (-2.5691, 50.6951) -> (-1.0691, 49.1951) centre (-1.0691, 50.6951) ccw projected
  line L2 (51.9309, 49.1951) -> (-1.0691, 49.1951) projected
  arc A3 (51.9309, 49.1951) -> (52.9309, 50.1951) centre (51.9309, 50.1951) ccw projected
  line L3 (52.9309, 77.1951) -> (52.9309, 50.1951) projected
  arc A4 (52.9309, 77.1951) -> (51.9309, 78.1951) centre (51.9309, 77.1951) ccw projected
  line L4 (-1.0691, 78.1951) -> (51.9309, 78.1951) projected
  arc A5 (-1.0691, 78.1951) -> (-2.5691, 76.6951) centre (-1.0691, 76.6951) ccw projected
  line L5 (-2.5691, 77.6365) -> (-2.5691, 76.6951) projected
  arc A6 (-1.6937, 79.2904) -> (-2.5691, 77.6365) centre (-0.5691, 77.6365) ccw projected
  line L6 (-1.6937, 79.2904) -> (4.1673, 83.2759) projected
  arc A7 (5.8543, 83.7951) -> (4.1673, 83.2759) centre (5.8543, 80.7951) ccw projected
  line L7 (5.8543, 83.7951) -> (50.1075, 83.7951) projected
  arc A8 (51.7945, 83.2759) -> (50.1075, 83.7951) centre (50.1075, 80.7951) ccw projected
  line L8 (51.7945, 83.2759) -> (57.2178, 79.588) projected
  arc A9 (58.5309, 77.1072) -> (57.2178, 79.588) centre (55.5309, 77.1072) ccw projected
  line L9 (58.5309, 77.1072) -> (58.5309, 50.283) projected
  arc A10 (57.2178, 47.8022) -> (58.5309, 50.283) centre (55.5309, 50.283) ccw projected
  line L10 (57.2178, 47.8022) -> (51.7945, 44.1143) projected
  arc A11 (50.1075, 43.5951) -> (51.7945, 44.1143) centre (50.1075, 46.5951) ccw projected
  line L11 (50.1075, 43.5951) -> (5.8543, 43.5951) projected
  circle A12 centre (6.4309, 80.9951) radius 1.35 projected
  circle A13 centre (28.4309, 80.9951) radius 1.35 projected
  circle A14 centre (55.7309, 74.6951) radius 1.35 projected
  circle A15 centre (6.4309, 46.3951) radius 1.35 projected
  circle A16 centre (28.4309, 46.3951) radius 1.35 projected
  circle A17 centre (55.7309, 52.6951) radius 1.35 projected
  circle A18 centre (50.4309, 80.9951) radius 1.35 projected
  circle A19 centre (50.4309, 46.3951) radius 1.35 projected
  arc A20 (-2.4691, 51.4697) -> (-1.0691, 49.0951) centre (-1.0691, 50.6951) ccw
  line L12 (-2.4691, 51.4697) -> (-2.4691, 49.7537)
  arc A21 (-2.4691, 49.7537) -> (-1.6375, 48.1826) centre (-0.5691, 49.7537) ccw
  line L13 (-1.6375, 48.1826) -> (4.2236, 44.197)
  arc A22 (4.2236, 44.197) -> (5.8543, 43.6951) centre (5.8543, 46.5951) ccw
  line L14 (5.8543, 43.6951) -> (50.1075, 43.6951)
  arc A23 (50.1075, 43.6951) -> (51.7382, 44.197) centre (50.1075, 46.5951) ccw
  line L15 (51.7382, 44.197) -> (57.1616, 47.8849)
  arc A24 (57.1616, 47.8849) -> (58.4309, 50.283) centre (55.5309, 50.283) ccw
  line L16 (58.4309, 50.283) -> (58.4309, 77.1072)
  arc A25 (58.4309, 77.1072) -> (57.1616, 79.5053) centre (55.5309, 77.1072) ccw
  line L17 (57.1616, 79.5053) -> (51.7382, 83.1932)
  arc A26 (51.7382, 83.1932) -> (50.1075, 83.6951) centre (50.1075, 80.7951) ccw
  line L18 (50.1075, 83.6951) -> (5.8543, 83.6951)
  arc A27 (5.8543, 83.6951) -> (4.2236, 83.1932) centre (5.8543, 80.7951) ccw
  line L19 (4.2236, 83.1932) -> (-1.6375, 79.2077)
  arc A28 (-1.6375, 79.2077) -> (-2.4691, 77.6365) centre (-0.5691, 77.6365) ccw
  line L20 (-2.4691, 77.6365) -> (-2.4691, 75.9205)
  arc A29 (-1.0691, 78.2951) -> (-2.4691, 75.9205) centre (-1.0691, 76.6951) ccw
  line L21 (-1.0691, 78.2951) -> (51.9309, 78.2951)
  arc A30 (53.0309, 77.1951) -> (51.9309, 78.2951) centre (51.9309, 77.1951) ccw
  line L22 (53.0309, 77.1951) -> (53.0309, 50.1951)
  arc A31 (51.9309, 49.0951) -> (53.0309, 50.1951) centre (51.9309, 50.1951) ccw
  line L23 (51.9309, 49.0951) -> (-1.0691, 49.0951)
  line L24 (-1.0691, 78.2951) -> (-1.0691, 49.0951)
  line L25 (-1.0691, 49.0951) -> (-3.0691, 49.0951)
  line L26 (-3.0691, 49.0951) -> (-3.0691, 78.2951)
  line L27 (-3.0691, 78.2951) -> (-1.0691, 78.2951)
  point P0 (11.501, 90.6951)
  dimension "d55" = 0.1
  dimension "d56" = 2
  constraints: 32 end point, 24 point on circle, 12 centre point, 2 parallel, 1 perpendicular, 23 other
  measures "d55" distance between parallel lines of L2 L23
  measures "d56" distance of L23.end L25.end
extrude "돌출8" cut sketch "스케치8" against normal blind 10 contours L25 L26 L27 A6 L5 A29 L20 A5 L24 A2 L12 A20 L1 A1 | A1 L1 A20 L12 A21 L25 | A21 L12 A20 L25 | A20 L12 A2 L1 | L1 A2 L12 A20 | L24 L2 A3 L3 A4 L4 L21 A30 L22 A31 L23 | A20 L12 A2 L24 | L24 L4 A4 L3 A3 L2 | L27 A28 L20 A29 L5 A6 | A5 L20 A29 L24 | L27 A29 L20 A28 | L20 A29 L5 A5 | A5 L5 A29 L20 | A12 | A13 | A15 | A16 | A18 | A19
sketch "스케치9" plane through (-11.501, -90.6951, 31.5) normal (0, 0, 1) x (1, 0, 0)
  circle A0 centre (28.4309, 80.9951) radius 1.35 projected
  circle A1 centre (6.4309, 46.3951) radius 1.35 projected
  circle A2 centre (50.4309, 80.9951) radius 1.35 projected
  circle A3 centre (6.4309, 80.9951) radius 1.35 projected
  circle A4 centre (28.4309, 46.3951) radius 1.35 projected
  circle A5 centre (50.4309, 46.3951) radius 1.35 projected
  arc A6 (51.9309, 49.0951) -> (53.0309, 50.1951) centre (51.9309, 50.1951) ccw projected
  line L0 (51.9309, 49.0951) -> (-3.0691, 49.0951) projected
  line L1 (-3.0691, 49.0951) -> (-3.0691, 78.2951) projected
  line L2 (-3.0691, 78.2951) -> (51.9309, 78.2951) projected
  arc A7 (53.0309, 77.1951) -> (51.9309, 78.2951) centre (51.9309, 77.1951) ccw projected
  line L3 (53.0309, 77.1951) -> (53.0309, 50.1951) projected
  line L4 (-2.399, 145.6951) -> (-2.399, 151.6951) projected
  line L5 (-2.399, 151.6951) -> (-11.399, 151.6951) projected
  line L6 (-11.399, 151.6951) -> (-11.399, 126.6951) projected
  line L7 (-11.399, 126.6951) -> (-17.399, 126.6951) projected
  line L8 (-17.399, 84.6951) -> (-17.399, 126.6951) projected
  line L9 (-11.399, 84.6951) -> (-17.399, 84.6951) projected
  line L10 (-11.399, 84.6951) -> (-11.399, 42.6951) projected
  line L11 (-11.399, 42.6951) -> (-17.399, 42.6951) projected
  line L12 (-17.399, 0.6951) -> (-17.399, 42.6951) projected
  line L13 (-11.399, 0.6951) -> (-17.399, 0.6951) projected
  line L14 (-11.399, 0.6951) -> (-11.399, -24.3049) projected
  line L15 (-11.399, -24.3049) -> (-2.399, -24.3049) projected
  line L16 (-2.399, -24.3049) -> (-2.399, -18.3049) projected
  line L17 (-2.399, -18.3049) -> (17.601, -18.3049) projected
  line L18 (17.601, -18.3049) -> (17.601, -24.3049) projected
  line L19 (17.601, -24.3049) -> (32.601, -24.3049) projected
  line L20 (32.601, -24.3049) -> (32.601, -18.3049) projected
  line L21 (32.601, -18.3049) -> (52.601, -18.3049) projected
  line L22 (52.601, -18.3049) -> (52.601, -24.3049) projected
  line L23 (52.601, -24.3049) -> (61.601, -24.3049) projected
  line L24 (61.601, -24.3049) -> (61.601, 0.6951) projected
  line L25 (61.601, 0.6951) -> (67.601, 0.6951) projected
  line L26 (67.601, 0.6951) -> (67.601, 42.6951) projected
  line L27 (67.601, 42.6951) -> (61.601, 42.6951) projected
  line L28 (61.601, 42.6951) -> (61.601, 84.6951) projected
  line L29 (61.601, 84.6951) -> (67.601, 84.6951) projected
  line L30 (67.601, 84.6951) -> (67.601, 126.6951) projected
  line L31 (67.601, 126.6951) -> (61.601, 126.6951) projected
  line L32 (61.601, 126.6951) -> (61.601, 151.6951) projected
  line L33 (61.601, 151.6951) -> (52.601, 151.6951) projected
  line L34 (52.601, 151.6951) -> (52.601, 145.6951) projected
  line L35 (52.601, 145.6951) -> (32.601, 145.6951) projected
  line L36 (32.601, 145.6951) -> (32.601, 151.6951) projected
  line L37 (32.601, 151.6951) -> (17.601, 151.6951) projected
  line L38 (17.601, 151.6951) -> (17.601, 145.6951) projected
  line L39 (17.601, 145.6951) -> (-2.399, 145.6951) projected
  line L40 (53.101, 99.8951) -> (49.101, 99.8951) projected
  arc A8 (48.101, 100.8951) -> (49.101, 99.8951) centre (48.101, 99.8951) ccw projected
  line L41 (48.101, 100.8951) -> (48.101, 126.4951) projected
  arc A9 (49.101, 127.4951) -> (48.101, 126.4951) centre (48.101, 127.4951) ccw projected
  line L42 (49.101, 127.4951) -> (53.1111, 127.4951) projected
  arc A10 (54.101, 126.6365) -> (53.1111, 127.4951) centre (54.101, 127.6365) ccw projected
  line L43 (54.101, 126.6365) -> (54.101, 100.8951) projected
  arc A11 (53.101, 99.8951) -> (54.101, 100.8951) centre (54.101, 99.8951) ccw projected
  arc A12 (0, 126.3951) -> (-1, 127.3951) centre (0, 127.3951) ccw projected
  line L44 (0, 126.3951) -> (0, 100.7951) projected
  arc A13 (-1, 99.7951) -> (0, 100.7951) centre (0, 99.7951) ccw projected
  line L45 (-1, 99.7951) -> (-5, 99.7951) projected
  arc A14 (-6, 100.7951) -> (-5, 99.7951) centre (-6, 99.7951) ccw projected
  line L46 (-6, 100.7951) -> (-6, 126.3951) projected
  arc A15 (-5, 127.3951) -> (-6, 126.3951) centre (-6, 127.3951) ccw projected
  line L47 (-5, 127.3951) -> (-1, 127.3951) projected
  line L48 (-6, 0.9951) -> (-6, 26.5951) projected
  arc A16 (-5, 27.5951) -> (-6, 26.5951) centre (-6, 27.5951) ccw projected
  line L49 (-5, 27.5951) -> (-1, 27.5951) projected
  arc A17 (0, 26.5951) -> (-1, 27.5951) centre (0, 27.5951) ccw projected
  line L50 (0, 26.5951) -> (0, 0.9951) projected
  arc A18 (-1, -0.0049) -> (0, 0.9951) centre (0, -0.0049) ccw projected
  line L51 (-1, -0.0049) -> (-5, -0.0049) projected
  arc A19 (-6, 0.9951) -> (-5, -0.0049) centre (-6, -0.0049) ccw projected
  line L52 (48.101, 0.8951) -> (48.101, 26.5951) projected
  arc A20 (49.096, 27.4951) -> (48.101, 26.5951) centre (48.101, 27.5951) ccw projected
  line L53 (49.096, 27.4951) -> (53.101, 27.4951) projected
  arc A21 (54.101, 26.4951) -> (53.101, 27.4951) centre (54.101, 27.4951) ccw projected
  line L54 (54.101, 26.4951) -> (54.101, 0.8951) projected
  arc A22 (53.101, -0.1049) -> (54.101, 0.8951) centre (54.101, -0.1049) ccw projected
  line L55 (53.101, -0.1049) -> (49.101, -0.1049) projected
  arc A23 (48.101, 0.8951) -> (49.101, -0.1049) centre (48.101, -0.1049) ccw projected
  line L56 (-17.399, 126.6951) -> (-11.399, 126.6951)
  line L57 (-11.399, 126.6951) -> (-11.399, 151.6951)
  line L58 (-11.399, 151.6951) -> (-17.399, 151.6951)
  line L59 (-17.399, 151.6951) -> (-17.399, 126.6951)
  line L60 (-17.399, 0.6951) -> (-11.399, 0.6951)
  line L61 (-11.399, 0.6951) -> (-11.399, -24.3049)
  line L62 (-11.399, -24.3049) -> (-17.399, -24.3049)
  line L63 (-17.399, -24.3049) -> (-17.399, 0.6951)
  line L64 (-17.399, 151.6951) -> (-17.399, -24.3049)
  line L65 (-17.399, -24.3049) -> (97.601, -24.3049)
  line L66 (97.601, -24.3049) -> (97.601, 151.6951)
  line L67 (97.601, 151.6951) -> (-17.399, 151.6951)
  point P0 (11.501, 90.6951)
  point P1 (97.601, 137.7581)
  point P2 (52.601, -24.3049)
  point P3 (-2.399, -24.3049)
  point P4 (-2.399, 151.6951)
  point P5 (52.601, 151.6951)
  point P6 (61.601, -24.3049)
  point P7 (61.601, 151.6951)
  constraints: 24 end point, 6 parallel, 3 perpendicular, 2 horizontal, 1 collinear, 1 other
extrude "돌출9" add sketch "스케치9" against normal up to surface (6 mm away) contours L4 L67 L38 L39 | L6 L7 L59 L58 | L67 L34 L35 L36 | L9 L10 L11 L64 | L67 L66 L65 L24 L25 L26 L27 L28 L29 L30 L31 L32 | L13 L14 L62 L63 | L65 L20 L21 L22 | L16 L17 L18 L65 | L40 A8 L41 A9 L42 A10 L43 A11 | L44 A13 L45 A14 L46 A15 L47 A12 | L48 A16 L49 A17 L50 A18 L51 A19 | L52 A20 L53 A21 L54 A22 L55 A23
sketch "스케치12" plane through (-11.501, -90.6951, 31.5) normal (0, 0, 1) x (1, 0, 0)
  spline S0 degree 3 poles (73.934, 13.3211) (73.4732, 13.3211) (72.9334, 13.3333) (72.3667, 13.461) (71.5295, 13.6498) (70.6997, 14.0808) (70.1984, 14.6743) (69.7907, 15.1568) (69.6309, 15.715) (69.6068, 16.2714) (69.6012, 16.3993) (69.601, 16.5269) (69.601, 16.6541) knots 0 0 0 0 0.252884 0.252884 0.252884 0.626442 0.626442 0.626442 0.930206 0.930206 0.930206 1 1 1 1 projected
  line L0 (86.268, 13.3211) -> (73.934, 13.3211) projected
  spline S1 degree 3 poles (90.601, 16.6541) (90.601, 16.1026) (90.5549, 15.5334) (90.2531, 15.0228) (89.8776, 14.3874) (89.1161, 13.8555) (88.289, 13.5846) (87.6852, 13.3869) (87.052, 13.3286) (86.5239, 13.3222) (86.4358, 13.3212) (86.3516, 13.3211) (86.268, 13.3211) knots 0 0 0 0 0.302665 0.302665 0.302665 0.679247 0.679247 0.679247 0.954138 0.954138 0.954138 1 1 1 1 projected
  line L1 (90.601, 107.3211) -> (90.601, 16.6541) projected
  arc A0 (90.601, 107.3211) -> (83.601, 114.3211) centre (83.601, 107.3211) ccw projected
  line L2 (76.601, 114.3211) -> (83.601, 114.3211) projected
  arc A1 (76.601, 114.3211) -> (69.601, 107.3211) centre (76.601, 107.3211) ccw projected
  line L3 (69.601, 16.6541) -> (69.601, 107.3211) projected
  circle A2 centre (28.4309, 80.9951) radius 1.35 projected
  circle A3 centre (6.4309, 46.3951) radius 1.35 projected
  circle A4 centre (50.4309, 80.9951) radius 1.35 projected
  circle A5 centre (6.4309, 80.9951) radius 1.35 projected
  circle A6 centre (28.4309, 46.3951) radius 1.35 projected
  circle A7 centre (50.4309, 46.3951) radius 1.35 projected
  arc A8 (51.9309, 49.0951) -> (53.0309, 50.1951) centre (51.9309, 50.1951) ccw projected
  line L4 (51.9309, 49.0951) -> (-3.0691, 49.0951) projected
  line L5 (-3.0691, 49.0951) -> (-3.0691, 78.2951) projected
  line L6 (-3.0691, 78.2951) -> (51.9309, 78.2951) projected
  arc A9 (53.0309, 77.1951) -> (51.9309, 78.2951) centre (51.9309, 77.1951) ccw projected
  line L7 (53.0309, 77.1951) -> (53.0309, 50.1951) projected
  line L8 (97.601, 151.6951) -> (-17.399, 151.6951) projected
  line L9 (-17.399, 151.6951) -> (-17.399, -24.3049) projected
  line L10 (-17.399, -24.3049) -> (97.601, -24.3049) projected
  line L11 (97.601, -24.3049) -> (97.601, 151.6951) projected
  line L12 (65.5418, -24.3049) -> (65.5418, 151.6951)
  line L13 (69.601, 28.9295) -> (65.5418, 28.9295)
  circle A10 centre (65.5418, 28.9295) radius 1.25
  line L14 (69.601, 95.7117) -> (65.5418, 95.7117)
  circle A11 centre (65.5418, 95.7117) radius 1.25
  line L15 (80.101, 13.3211) -> (80.101, 7.3211)
  line L16 (80.101, 13.3211) -> (86.101, 13.3211) construction
  circle A12 centre (80.101, 7.3211) radius 1.25
  line L17 (81.351, 114.3211) -> (81.351, 120.3211)
  circle A13 centre (81.351, 120.3211) radius 1.25
  point P0 (11.501, 90.6951)
  dimension "d69" = 2.5
  dimension "d70" = 2.5
  dimension "d71" = 6
  dimension "d72" = 90
  dimension "d73" = 2.5
  dimension "d74" = 6
  dimension "d75" = 2.5
  constraints: 12 end point, 7 point on line, 4 centre point, 4 coincident, 4 perpendicular, 2 vertical, 1 horizontal, 1 midpoint
  measures "d69" diameter of A10
  measures "d70" diameter of A11
  measures "d71" distance of L15.start L15.end
  measures "d72" angle of L15 L16
  measures "d73" diameter of A12
  measures "d74" distance of L17.start L17.end
  measures "d75" diameter of A13
extrude "돌출12" cut sketch "스케치12" against normal blind 10 contours A10 L12 L13 | L13 L12 A10 | A11 L12 L14 | L14 L12 A11 | L12 A10 | L12 A11 | A12 | A13
